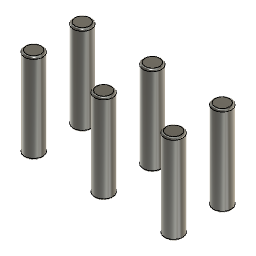
_Pins for Outer Cover.100f071b-10c4-4fbe-a039-9e613c86b4a1 (Autodesk Fusion 360 design; units mm, degrees)
Autodesk Fusion 360 part; units mm, degrees
sketch "Sketch1" plane through (0, 0, 0) normal (0, 0, 1) x (1, 0, 0)
  circle A0 centre (0, 0) radius 1.475
  circle A1 centre (11.5, 0) radius 1.475
  circle A2 centre (23, 0) radius 1.475
  circle A3 centre (0, 8) radius 1.475
  circle A4 centre (11.5, 8) radius 1.475
  circle A5 centre (23, 8) radius 1.475
  dimension "d2" = 2.95
  dimension "d5" = 23
  dimension "d6" = 8
  constraint coincident A0.centre origin
  measures "d2" diameter of A0
extrude "Extrude1" add sketch "Sketch1" along normal blind 14.7 makes body 1 at (24.4732, -0.0735, 9.8) makes body 2 at (12.9732, 7.9265, 9.8) makes body 3 at (1.4732, -0.0735, 9.8) makes body 4 at (24.4732, 7.9265, 9.8) makes body 5 at (12.9732, -0.0735, 9.8) makes body 6 at (1.4732, 7.9265, 9.8)
fillet "Fillet1" radius 0.3 12 edges at (21.6248, -0.5334, 0) (21.6248, -0.5334, 14.7) (10.1248, 7.4666, 14.7) (10.1248, 7.4666, 0) (-1.3752, -0.5334, 0) (-1.3752, -0.5334, 14.7) (21.6248, 7.4666, 14.7) (21.6248, 7.4666, 0) (10.1248, -0.5334, 0) (10.1248, -0.5334, 14.7) (-1.3752, 7.4666, 14.7) (-1.3752, 7.4666, 0) on bodies 1 2 3 4 5 6
